Autodesk Fusion 360 part; units mm, degrees
note: some values were not read from the file. Chosen so that the rebuilt part matches the saved one: which bodies a step acts on; which face or edge a step refers to. Set by a fixed rule: which sketch regions a step uses.
(part 3 of 3)
sketch "Sketch1" plane through (0, 0, 0) normal (0, 0, 1) x (1, 0, 0)
  line L0 (-92, 39) -> (92, 39)
  line L1 (92, 39) -> (92, -39)
  line L2 (92, -39) -> (-92, -39)
  line L3 (-92, -39) -> (-92, 39)
  line L4 (-92, 39) -> (92, -39) construction
  line L5 (92, 39) -> (-92, -39) construction
  dimension "d1" = 184
  dimension "d2" = 78
  constraint horizontal L0
  constraint perpendicular L0 L1
  constraint parallel L0 L2
  constraint parallel L1 L3
  constraint coincident L4 origin
  constraint coincident L5 origin
  measures "d1" distance of L1.end L2.end
  measures "d2" distance of L0.end L1.end
extrude "Extrude1" add sketch "Sketch1" along normal blind 6
sketch "Sketch2" plane through (0, 0, 6) normal (0, 0, 1) x (-1, 0, 0)
  line L0 (92, 39) -> (-92, 39)
  line L1 (-92, 39) -> (-92, -39)
  line L2 (-92, -39) -> (92, -39)
  line L3 (92, -39) -> (92, 39)
  line L4 (87, -34) -> (81, -34)
  line L5 (81, -34) -> (81, -29)
  line L6 (81, -29) -> (87, -29)
  line L7 (87, -29) -> (87, -34)
  dimension "d5" = 6
  dimension "d6" = 5
  constraint horizontal L4
  constraint vertical L5
  constraint horizontal L6
  constraint vertical L7
  measures "d5" distance of L4.start L4.end
  measures "d6" distance of L4.start L6.end
extrude "Extrude2" cut sketch "Sketch2" against normal blind 6 contours L4 L5 L6 L7
pattern_linear "R-Pattern1" count 6 spacing 12.6 along (0, -1, 0) count 6 spacing 33.4 along (1, 0, 0) of "Extrude2"
sketch "Sketch3" plane through (0, 0, 6) normal (0, 0, 1) x (-1, 0, 0)
  line L0 (-86, 29) -> (-86, 34)
  line L1 (-86, 34) -> (-80, 34)
  line L2 (-80, 34) -> (-80, 29)
  line L3 (-80, 29) -> (-86, 29)
  line L4 (-86, 16.4) -> (-86, 21.4)
  line L5 (-86, 21.4) -> (-80, 21.4)
  line L6 (-80, 21.4) -> (-80, 16.4)
  line L7 (-80, 16.4) -> (-86, 16.4)
  line L8 (-86, 3.8) -> (-86, 8.8)
  line L9 (-86, 8.8) -> (-80, 8.8)
  line L10 (-80, 8.8) -> (-80, 3.8)
  line L11 (-80, 3.8) -> (-86, 3.8)
  line L12 (-86, -8.8) -> (-86, -3.8)
  line L13 (-86, -3.8) -> (-80, -3.8)
  line L14 (-80, -3.8) -> (-80, -8.8)
  line L15 (-80, -8.8) -> (-86, -8.8)
  line L16 (-86, -21.4) -> (-86, -16.4)
  line L17 (-86, -16.4) -> (-80, -16.4)
  line L18 (-80, -16.4) -> (-80, -21.4)
  line L19 (-80, -21.4) -> (-86, -21.4)
  line L20 (-86, -34) -> (-86, -29)
  line L21 (-86, -29) -> (-80, -29)
  line L22 (-80, -29) -> (-80, -34)
  line L23 (-80, -34) -> (-86, -34)
  line L24 (-52.6, 29) -> (-52.6, 34)
  line L25 (-52.6, 34) -> (-46.6, 34)
  line L26 (-46.6, 34) -> (-46.6, 29)
  line L27 (-46.6, 29) -> (-52.6, 29)
  line L28 (-52.6, 16.4) -> (-52.6, 21.4)
  line L29 (-52.6, 21.4) -> (-46.6, 21.4)
  line L30 (-46.6, 21.4) -> (-46.6, 16.4)
  line L31 (-46.6, 16.4) -> (-52.6, 16.4)
  line L32 (-52.6, 3.8) -> (-52.6, 8.8)
  line L33 (-52.6, 8.8) -> (-46.6, 8.8)
  line L34 (-46.6, 8.8) -> (-46.6, 3.8)
  line L35 (-46.6, 3.8) -> (-52.6, 3.8)
  line L36 (-52.6, -8.8) -> (-52.6, -3.8)
  line L37 (-52.6, -3.8) -> (-46.6, -3.8)
  line L38 (-46.6, -3.8) -> (-46.6, -8.8)
  line L39 (-46.6, -8.8) -> (-52.6, -8.8)
  line L40 (-52.6, -21.4) -> (-52.6, -16.4)
  line L41 (-52.6, -16.4) -> (-46.6, -16.4)
  line L42 (-46.6, -16.4) -> (-46.6, -21.4)
  line L43 (-46.6, -21.4) -> (-52.6, -21.4)
  line L44 (-52.6, -34) -> (-52.6, -29)
  line L45 (-52.6, -29) -> (-46.6, -29)
  line L46 (-46.6, -29) -> (-46.6, -34)
  line L47 (-46.6, -34) -> (-52.6, -34)
  line L48 (-19.2, 29) -> (-19.2, 34)
  line L49 (-19.2, 34) -> (-13.2, 34)
  line L50 (-13.2, 34) -> (-13.2, 29)
  line L51 (-13.2, 29) -> (-19.2, 29)
  line L52 (-19.2, 16.4) -> (-19.2, 21.4)
  line L53 (-19.2, 21.4) -> (-13.2, 21.4)
  line L54 (-13.2, 21.4) -> (-13.2, 16.4)
  line L55 (-13.2, 16.4) -> (-19.2, 16.4)
  line L56 (-19.2, 3.8) -> (-19.2, 8.8)
  line L57 (-19.2, 8.8) -> (-13.2, 8.8)
  line L58 (-13.2, 8.8) -> (-13.2, 3.8)
  line L59 (-13.2, 3.8) -> (-19.2, 3.8)
  line L60 (-19.2, -8.8) -> (-19.2, -3.8)
  line L61 (-19.2, -3.8) -> (-13.2, -3.8)
  line L62 (-13.2, -3.8) -> (-13.2, -8.8)
  line L63 (-13.2, -8.8) -> (-19.2, -8.8)
  line L64 (-19.2, -21.4) -> (-19.2, -16.4)
  line L65 (-19.2, -16.4) -> (-13.2, -16.4)
  line L66 (-13.2, -16.4) -> (-13.2, -21.4)
  line L67 (-13.2, -21.4) -> (-19.2, -21.4)
  line L68 (-19.2, -34) -> (-19.2, -29)
  line L69 (-19.2, -29) -> (-13.2, -29)
  line L70 (-13.2, -29) -> (-13.2, -34)
  line L71 (-13.2, -34) -> (-19.2, -34)
  line L72 (14.2, 29) -> (14.2, 34)
  line L73 (14.2, 34) -> (20.2, 34)
  line L74 (20.2, 34) -> (20.2, 29)
  line L75 (20.2, 29) -> (14.2, 29)
  line L76 (14.2, 16.4) -> (14.2, 21.4)
  line L77 (14.2, 21.4) -> (20.2, 21.4)
  line L78 (20.2, 21.4) -> (20.2, 16.4)
  line L79 (20.2, 16.4) -> (14.2, 16.4)
  line L80 (14.2, 3.8) -> (14.2, 8.8)
  line L81 (14.2, 8.8) -> (20.2, 8.8)
  line L82 (20.2, 8.8) -> (20.2, 3.8)
  line L83 (20.2, 3.8) -> (14.2, 3.8)
  line L84 (14.2, -8.8) -> (14.2, -3.8)
  line L85 (14.2, -3.8) -> (20.2, -3.8)
  line L86 (20.2, -3.8) -> (20.2, -8.8)
  line L87 (20.2, -8.8) -> (14.2, -8.8)
  line L88 (14.2, -21.4) -> (14.2, -16.4)
  line L89 (14.2, -16.4) -> (20.2, -16.4)
  line L90 (20.2, -16.4) -> (20.2, -21.4)
  line L91 (20.2, -21.4) -> (14.2, -21.4)
  line L92 (14.2, -34) -> (14.2, -29)
  line L93 (14.2, -29) -> (20.2, -29)
  line L94 (20.2, -29) -> (20.2, -34)
  line L95 (20.2, -34) -> (14.2, -34)
  line L96 (47.6, 29) -> (47.6, 34)
  line L97 (47.6, 34) -> (53.6, 34)
  line L98 (53.6, 34) -> (53.6, 29)
  line L99 (53.6, 29) -> (47.6, 29)
  line L100 (47.6, 16.4) -> (47.6, 21.4)
  line L101 (47.6, 21.4) -> (53.6, 21.4)
  line L102 (53.6, 21.4) -> (53.6, 16.4)
  line L103 (53.6, 16.4) -> (47.6, 16.4)
  line L104 (47.6, 3.8) -> (47.6, 8.8)
  line L105 (47.6, 8.8) -> (53.6, 8.8)
  line L106 (53.6, 8.8) -> (53.6, 3.8)
  line L107 (53.6, 3.8) -> (47.6, 3.8)
  line L108 (47.6, -8.8) -> (47.6, -3.8)
  line L109 (47.6, -3.8) -> (53.6, -3.8)
  line L110 (53.6, -3.8) -> (53.6, -8.8)
  line L111 (53.6, -8.8) -> (47.6, -8.8)
  line L112 (47.6, -21.4) -> (47.6, -16.4)
  line L113 (47.6, -16.4) -> (53.6, -16.4)
  line L114 (53.6, -16.4) -> (53.6, -21.4)
  line L115 (53.6, -21.4) -> (47.6, -21.4)
  line L116 (47.6, -34) -> (47.6, -29)
  line L117 (47.6, -29) -> (53.6, -29)
  line L118 (53.6, -29) -> (53.6, -34)
  line L119 (53.6, -34) -> (47.6, -34)
  line L120 (81, 29) -> (81, 34)
  line L121 (81, 34) -> (87, 34)
  line L122 (87, 34) -> (87, 29)
  line L123 (87, 29) -> (81, 29)
  line L124 (81, 16.4) -> (81, 21.4)
  line L125 (81, 21.4) -> (87, 21.4)
  line L126 (87, 21.4) -> (87, 16.4)
  line L127 (87, 16.4) -> (81, 16.4)
  line L128 (81, 3.8) -> (81, 8.8)
  line L129 (81, 8.8) -> (87, 8.8)
  line L130 (87, 8.8) -> (87, 3.8)
  line L131 (87, 3.8) -> (81, 3.8)
  line L132 (81, -8.8) -> (81, -3.8)
  line L133 (81, -3.8) -> (87, -3.8)
  line L134 (87, -3.8) -> (87, -8.8)
  line L135 (87, -8.8) -> (81, -8.8)
  line L136 (81, -21.4) -> (81, -16.4)
  line L137 (81, -16.4) -> (87, -16.4)
  line L138 (87, -16.4) -> (87, -21.4)
  line L139 (87, -21.4) -> (81, -21.4)
  line L140 (81, -34) -> (81, -29)
  line L141 (81, -29) -> (87, -29)
  line L142 (87, -29) -> (87, -34)
  line L143 (87, -34) -> (81, -34)
  line L144 (92, 39) -> (-92, 39)
  line L145 (-92, 39) -> (-92, -39)
  line L146 (-92, -39) -> (92, -39)
  line L147 (92, -39) -> (92, 39)
  line L148 (53.6, -34) -> (81, -34) construction
  line L149 (67.3, -34) -> (67.3, 39) construction
  line L150 (70, -34) -> (65, -34)
  line L151 (65, -34) -> (65, -28)
  line L152 (65, -28) -> (70, -28)
  line L153 (70, -28) -> (70, -34)
  dimension "d13" = 6
  dimension "d14" = 5
  constraint coincident L118.end L119.start
  constraint coincident L140.start L143.end
  constraint midpoint L148 L149.start
  constraint coincident L144 L149.end
  constraint perpendicular L144 L149
  constraint horizontal L150
  constraint vertical L151
  constraint horizontal L152
  constraint vertical L153
  constraint coincident L148 L150.start
  measures "d13" distance of L150.start L152.end
  measures "d14" distance of L151 L153
extrude "Extrude3" cut sketch "Sketch3" against normal blind 6 contours L150 L151 L152 L153
pattern_linear "R-Pattern2" count 5 spacing 15.5 along (0, -1, 0) count 5 spacing 33.75 along (1, 0, 0) of "Extrude3"
fillet "Fillet1" radius 3 1 edges at (-92, -39, 3)
fillet "Fillet1" radius 3 3 edges at (-92, 39, 3) (92, 39, 3) (92, -39, 3)
sketch "Sketch4" plane through (0, 0, 6) normal (0, 0, 1) x (-1, 0, 0)
  line L0 (-70, 28) -> (-70, 34)
  line L1 (-70, 34) -> (-65, 34)
  line L2 (-65, 34) -> (-65, 28)
  line L3 (-65, 28) -> (-70, 28)
  line L4 (-70, 12.5) -> (-70, 18.5)
  line L5 (-70, 18.5) -> (-65, 18.5)
  line L6 (-65, 18.5) -> (-65, 12.5)
  line L7 (-65, 12.5) -> (-70, 12.5)
  line L8 (-70, -3) -> (-70, 3)
  line L9 (-70, 3) -> (-65, 3)
  line L10 (-65, 3) -> (-65, -3)
  line L11 (-65, -3) -> (-70, -3)
  line L12 (-70, -18.5) -> (-70, -12.5)
  line L13 (-70, -12.5) -> (-65, -12.5)
  line L14 (-65, -12.5) -> (-65, -18.5)
  line L15 (-65, -18.5) -> (-70, -18.5)
  line L16 (-70, -34) -> (-70, -28)
  line L17 (-70, -28) -> (-65, -28)
  line L18 (-65, -28) -> (-65, -34)
  line L19 (-65, -34) -> (-70, -34)
  line L20 (-36.25, 28) -> (-36.25, 34)
  line L21 (-36.25, 34) -> (-31.25, 34)
  line L22 (-31.25, 34) -> (-31.25, 28)
  line L23 (-31.25, 28) -> (-36.25, 28)
  line L24 (-36.25, 12.5) -> (-36.25, 18.5)
  line L25 (-36.25, 18.5) -> (-31.25, 18.5)
  line L26 (-31.25, 18.5) -> (-31.25, 12.5)
  line L27 (-31.25, 12.5) -> (-36.25, 12.5)
  line L28 (-36.25, -3) -> (-36.25, 3)
  line L29 (-36.25, 3) -> (-31.25, 3)
  line L30 (-31.25, 3) -> (-31.25, -3)
  line L31 (-31.25, -3) -> (-36.25, -3)
  line L32 (-36.25, -18.5) -> (-36.25, -12.5)
  line L33 (-36.25, -12.5) -> (-31.25, -12.5)
  line L34 (-31.25, -12.5) -> (-31.25, -18.5)
  line L35 (-31.25, -18.5) -> (-36.25, -18.5)
  line L36 (-36.25, -34) -> (-36.25, -28)
  line L37 (-36.25, -28) -> (-31.25, -28)
  line L38 (-31.25, -28) -> (-31.25, -34)
  line L39 (-31.25, -34) -> (-36.25, -34)
  line L40 (-2.5, 28) -> (-2.5, 34)
  line L41 (-2.5, 34) -> (2.5, 34)
  line L42 (2.5, 34) -> (2.5, 28)
  line L43 (2.5, 28) -> (-2.5, 28)
  line L44 (-2.5, 12.5) -> (-2.5, 18.5)
  line L45 (-2.5, 18.5) -> (2.5, 18.5)
  line L46 (2.5, 18.5) -> (2.5, 12.5)
  line L47 (2.5, 12.5) -> (-2.5, 12.5)
  line L48 (-2.5, -3) -> (-2.5, 3)
  line L49 (-2.5, 3) -> (2.5, 3)
  line L50 (2.5, 3) -> (2.5, -3)
  line L51 (2.5, -3) -> (-2.5, -3)
  line L52 (-2.5, -18.5) -> (-2.5, -12.5)
  line L53 (-2.5, -12.5) -> (2.5, -12.5)
  line L54 (2.5, -12.5) -> (2.5, -18.5)
  line L55 (2.5, -18.5) -> (-2.5, -18.5)
  line L56 (-2.5, -34) -> (-2.5, -28)
  line L57 (-2.5, -28) -> (2.5, -28)
  line L58 (2.5, -28) -> (2.5, -34)
  line L59 (2.5, -34) -> (-2.5, -34)
  line L60 (31.25, 28) -> (31.25, 34)
  line L61 (31.25, 34) -> (36.25, 34)
  line L62 (36.25, 34) -> (36.25, 28)
  line L63 (36.25, 28) -> (31.25, 28)
  line L64 (31.25, 12.5) -> (31.25, 18.5)
  line L65 (31.25, 18.5) -> (36.25, 18.5)
  line L66 (36.25, 18.5) -> (36.25, 12.5)
  line L67 (36.25, 12.5) -> (31.25, 12.5)
  line L68 (31.25, -3) -> (31.25, 3)
  line L69 (31.25, 3) -> (36.25, 3)
  line L70 (36.25, 3) -> (36.25, -3)
  line L71 (36.25, -3) -> (31.25, -3)
  line L72 (31.25, -18.5) -> (31.25, -12.5)
  line L73 (31.25, -12.5) -> (36.25, -12.5)
  line L74 (36.25, -12.5) -> (36.25, -18.5)
  line L75 (36.25, -18.5) -> (31.25, -18.5)
  line L76 (31.25, -34) -> (31.25, -28)
  line L77 (31.25, -28) -> (36.25, -28)
  line L78 (36.25, -28) -> (36.25, -34)
  line L79 (36.25, -34) -> (31.25, -34)
  line L80 (65, 28) -> (65, 34)
  line L81 (65, 34) -> (70, 34)
  line L82 (70, 34) -> (70, 28)
  line L83 (70, 28) -> (65, 28)
  line L84 (65, 12.5) -> (65, 18.5)
  line L85 (65, 18.5) -> (70, 18.5)
  line L86 (70, 18.5) -> (70, 12.5)
  line L87 (70, 12.5) -> (65, 12.5)
  line L88 (65, -3) -> (65, 3)
  line L89 (65, 3) -> (70, 3)
  line L90 (70, 3) -> (70, -3)
  line L91 (70, -3) -> (65, -3)
  line L92 (65, -18.5) -> (65, -12.5)
  line L93 (65, -12.5) -> (70, -12.5)
  line L94 (70, -12.5) -> (70, -18.5)
  line L95 (70, -18.5) -> (65, -18.5)
  line L96 (65, -34) -> (65, -28)
  line L97 (65, -28) -> (70, -28)
  line L98 (70, -28) -> (70, -34)
  line L99 (70, -34) -> (65, -34)
  line L100 (-86, 29) -> (-86, 34)
  line L101 (-86, 34) -> (-80, 34)
  line L102 (-80, 34) -> (-80, 29)
  line L103 (-80, 29) -> (-86, 29)
  line L104 (-86, 16.4) -> (-86, 21.4)
  line L105 (-86, 21.4) -> (-80, 21.4)
  line L106 (-80, 21.4) -> (-80, 16.4)
  line L107 (-80, 16.4) -> (-86, 16.4)
  line L108 (-86, 3.8) -> (-86, 8.8)
  line L109 (-86, 8.8) -> (-80, 8.8)
  line L110 (-80, 8.8) -> (-80, 3.8)
  line L111 (-80, 3.8) -> (-86, 3.8)
  line L112 (-86, -8.8) -> (-86, -3.8)
  line L113 (-86, -3.8) -> (-80, -3.8)
  line L114 (-80, -3.8) -> (-80, -8.8)
  line L115 (-80, -8.8) -> (-86, -8.8)
  line L116 (-86, -21.4) -> (-86, -16.4)
  line L117 (-86, -16.4) -> (-80, -16.4)
  line L118 (-80, -16.4) -> (-80, -21.4)
  line L119 (-80, -21.4) -> (-86, -21.4)
  line L120 (-86, -34) -> (-86, -29)
  line L121 (-86, -29) -> (-80, -29)
  line L122 (-80, -29) -> (-80, -34)
  line L123 (-80, -34) -> (-86, -34)
  line L124 (-52.6, 29) -> (-52.6, 34)
  line L125 (-52.6, 34) -> (-46.6, 34)
  line L126 (-46.6, 34) -> (-46.6, 29)
  line L127 (-46.6, 29) -> (-52.6, 29)
  line L128 (-52.6, 16.4) -> (-52.6, 21.4)
  line L129 (-52.6, 21.4) -> (-46.6, 21.4)
  line L130 (-46.6, 21.4) -> (-46.6, 16.4)
  line L131 (-46.6, 16.4) -> (-52.6, 16.4)
  line L132 (-52.6, 3.8) -> (-52.6, 8.8)
  line L133 (-52.6, 8.8) -> (-46.6, 8.8)
  line L134 (-46.6, 8.8) -> (-46.6, 3.8)
  line L135 (-46.6, 3.8) -> (-52.6, 3.8)
  line L136 (-52.6, -8.8) -> (-52.6, -3.8)
  line L137 (-52.6, -3.8) -> (-46.6, -3.8)
  line L138 (-46.6, -3.8) -> (-46.6, -8.8)
  line L139 (-46.6, -8.8) -> (-52.6, -8.8)
  line L140 (-52.6, -21.4) -> (-52.6, -16.4)
  line L141 (-52.6, -16.4) -> (-46.6, -16.4)
  line L142 (-46.6, -16.4) -> (-46.6, -21.4)
  line L143 (-46.6, -21.4) -> (-52.6, -21.4)
  line L144 (-52.6, -34) -> (-52.6, -29)
  line L145 (-52.6, -29) -> (-46.6, -29)
  line L146 (-46.6, -29) -> (-46.6, -34)
  line L147 (-46.6, -34) -> (-52.6, -34)
  line L148 (-19.2, 29) -> (-19.2, 34)
  line L149 (-19.2, 34) -> (-13.2, 34)
  line L150 (-13.2, 34) -> (-13.2, 29)
  line L151 (-13.2, 29) -> (-19.2, 29)
  line L152 (-19.2, 16.4) -> (-19.2, 21.4)
  line L153 (-19.2, 21.4) -> (-13.2, 21.4)
  line L154 (-13.2, 21.4) -> (-13.2, 16.4)
  line L155 (-13.2, 16.4) -> (-19.2, 16.4)
  line L156 (-19.2, 3.8) -> (-19.2, 8.8)
  line L157 (-19.2, 8.8) -> (-13.2, 8.8)
  line L158 (-13.2, 8.8) -> (-13.2, 3.8)
  line L159 (-13.2, 3.8) -> (-19.2, 3.8)
  line L160 (-19.2, -8.8) -> (-19.2, -3.8)
  line L161 (-19.2, -3.8) -> (-13.2, -3.8)
  line L162 (-13.2, -3.8) -> (-13.2, -8.8)
  line L163 (-13.2, -8.8) -> (-19.2, -8.8)
  line L164 (-19.2, -21.4) -> (-19.2, -16.4)
  line L165 (-19.2, -16.4) -> (-13.2, -16.4)
  line L166 (-13.2, -16.4) -> (-13.2, -21.4)
  line L167 (-13.2, -21.4) -> (-19.2, -21.4)
  line L168 (-19.2, -34) -> (-19.2, -29)
  line L169 (-19.2, -29) -> (-13.2, -29)
  line L170 (-13.2, -29) -> (-13.2, -34)
  line L171 (-13.2, -34) -> (-19.2, -34)
  line L172 (14.2, 29) -> (14.2, 34)
  line L173 (14.2, 34) -> (20.2, 34)
  line L174 (20.2, 34) -> (20.2, 29)
  line L175 (20.2, 29) -> (14.2, 29)
  line L176 (14.2, 16.4) -> (14.2, 21.4)
  line L177 (14.2, 21.4) -> (20.2, 21.4)
  line L178 (20.2, 21.4) -> (20.2, 16.4)
  line L179 (20.2, 16.4) -> (14.2, 16.4)
  line L180 (14.2, 3.8) -> (14.2, 8.8)
  line L181 (14.2, 8.8) -> (20.2, 8.8)
  line L182 (20.2, 8.8) -> (20.2, 3.8)
  line L183 (20.2, 3.8) -> (14.2, 3.8)
  line L184 (14.2, -8.8) -> (14.2, -3.8)
  line L185 (14.2, -3.8) -> (20.2, -3.8)
  line L186 (20.2, -3.8) -> (20.2, -8.8)
  line L187 (20.2, -8.8) -> (14.2, -8.8)
  line L188 (14.2, -21.4) -> (14.2, -16.4)
  line L189 (14.2, -16.4) -> (20.2, -16.4)
  line L190 (20.2, -16.4) -> (20.2, -21.4)
  line L191 (20.2, -21.4) -> (14.2, -21.4)
  line L192 (14.2, -34) -> (14.2, -29)
  line L193 (14.2, -29) -> (20.2, -29)
  line L194 (20.2, -29) -> (20.2, -34)
  line L195 (20.2, -34) -> (14.2, -34)
  line L196 (47.6, 29) -> (47.6, 34)
  line L197 (47.6, 34) -> (53.6, 34)
  line L198 (53.6, 34) -> (53.6, 29)
  line L199 (53.6, 29) -> (47.6, 29)
  line L200 (47.6, 16.4) -> (47.6, 21.4)
  line L201 (47.6, 21.4) -> (53.6, 21.4)
  line L202 (53.6, 21.4) -> (53.6, 16.4)
  line L203 (53.6, 16.4) -> (47.6, 16.4)
  line L204 (47.6, 3.8) -> (47.6, 8.8)
  line L205 (47.6, 8.8) -> (53.6, 8.8)
  line L206 (53.6, 8.8) -> (53.6, 3.8)
  line L207 (53.6, 3.8) -> (47.6, 3.8)
  line L208 (47.6, -8.8) -> (47.6, -3.8)
  line L209 (47.6, -3.8) -> (53.6, -3.8)
  line L210 (53.6, -3.8) -> (53.6, -8.8)
  line L211 (53.6, -8.8) -> (47.6, -8.8)
  line L212 (47.6, -21.4) -> (47.6, -16.4)
  line L213 (47.6, -16.4) -> (53.6, -16.4)
  line L214 (53.6, -16.4) -> (53.6, -21.4)
  line L215 (53.6, -21.4) -> (47.6, -21.4)
  line L216 (47.6, -34) -> (47.6, -29)
  line L217 (47.6, -29) -> (53.6, -29)
  line L218 (53.6, -29) -> (53.6, -34)
  line L219 (53.6, -34) -> (47.6, -34)
  line L220 (81, 29) -> (81, 34)
  line L221 (81, 34) -> (87, 34)
  line L222 (87, 34) -> (87, 29)
  line L223 (87, 29) -> (81, 29)
  line L224 (81, 16.4) -> (81, 21.4)
  line L225 (81, 21.4) -> (87, 21.4)
  line L226 (87, 21.4) -> (87, 16.4)
  line L227 (87, 16.4) -> (81, 16.4)
  line L228 (81, 3.8) -> (81, 8.8)
  line L229 (81, 8.8) -> (87, 8.8)
  line L230 (87, 8.8) -> (87, 3.8)
  line L231 (87, 3.8) -> (81, 3.8)
  line L232 (81, -8.8) -> (81, -3.8)
  line L233 (81, -3.8) -> (87, -3.8)
  line L234 (87, -3.8) -> (87, -8.8)
  line L235 (87, -8.8) -> (81, -8.8)
  line L236 (81, -21.4) -> (81, -16.4)
  line L237 (81, -16.4) -> (87, -16.4)
  line L238 (87, -16.4) -> (87, -21.4)
  line L239 (87, -21.4) -> (81, -21.4)
  line L240 (81, -34) -> (81, -29)
  line L241 (81, -29) -> (87, -29)
  line L242 (87, -29) -> (87, -34)
  line L243 (87, -34) -> (81, -34)
  arc A0 (-89, 39) -> (-92, 36) centre (-89, 36) ccw
  line L244 (-92, 36) -> (-92, -36)
  arc A1 (-92, -36) -> (-89, -39) centre (-89, -36) ccw
  line L245 (-89, -39) -> (89, -39)
  arc A2 (89, -39) -> (92, -36) centre (89, -36) ccw
  line L246 (92, -36) -> (92, 36)
  arc A3 (92, 36) -> (89, 39) centre (89, 36) ccw
  line L247 (89, 39) -> (-89, 39)

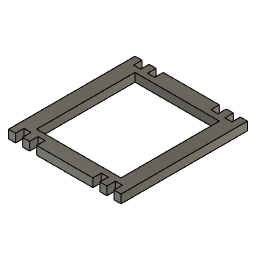
design "Carrier Top Piece"
Autodesk Fusion 360 part; units mm, degrees
sketch "Sketch1" plane through (0, 0, 0) normal (0, 0, 1) x (1, 0, 0)
  line L0 (40, 45) -> (-40, 45)
  line L1 (-40, 45) -> (-40, -45)
  line L2 (-40, -45) -> (40, -45)
  line L3 (40, -45) -> (40, 45)
  line L4 (40, 45) -> (-40, -45) construction
  line L5 (-40, 45) -> (40, -45) construction
  line L6 (30, 35) -> (-30, 35)
  line L7 (-30, 35) -> (-30, -35)
  line L8 (-30, -35) -> (30, -35)
  line L9 (30, -35) -> (30, 35)
  line L10 (30, 35) -> (-30, -35) construction
  line L11 (-30, 35) -> (30, -35) construction
  dimension "d1" = 80
  dimension "d2" = 90
  dimension "d3" = 60
  dimension "d6" = 10
  constraint horizontal L0
  constraint perpendicular L0 L1
  constraint parallel L0 L2
  constraint parallel L1 L3
  constraint coincident L4 origin
  constraint coincident L5 origin
  constraint horizontal L6
  constraint perpendicular L6 L7
  constraint parallel L6 L8
  constraint parallel L7 L9
  constraint coincident L10 origin
  constraint coincident L11 origin
  measures "d1" distance of L1.end L2.end
  measures "d2" distance of L0.end L1.end
  measures "d3" distance of L7.end L8.end
  measures "d6" distance of L0 L6
extrude "Extrude1" add sketch "Sketch1" along normal blind 6
sketch "Sketch2" plane through (0, 0, 6) normal (0, 0, 1) x (-1, 0, 0)
  line L0 (-30, -35) -> (-30, 35)
  line L1 (-30, 35) -> (30, 35)
  line L2 (30, 35) -> (30, -35)
  line L3 (30, -35) -> (-30, -35)
  line L4 (-40, 45) -> (-40, -45)
  line L5 (-40, -45) -> (40, -45)
  line L6 (40, -45) -> (40, 45)
  line L7 (40, 45) -> (-40, 45)
  line L8 (-40, 45) -> (-35, 45) construction
  line L9 (-35, 45) -> (-35, 39) construction
  line L10 (-35, 39) -> (-40, 39) construction
  line L11 (-40, 39) -> (-40, 45) construction
  line L12 (-35, 45) -> (-30, 45) construction
  line L13 (-30, 45) -> (-30, 39) construction
  line L14 (-30, 39) -> (-35, 39) construction
  line L15 (-35, 39) -> (-35, 45) construction
  line L16 (-30, 45) -> (-25, 45) construction
  line L17 (-25, 45) -> (-25, 39) construction
  line L18 (-25, 39) -> (-30, 39) construction
  line L19 (-30, 39) -> (-30, 45) construction
  line L20 (-25, 45) -> (-20, 45) construction
  line L21 (-20, 45) -> (-20, 39) construction
  line L22 (-20, 39) -> (-25, 39) construction
  line L23 (-25, 39) -> (-25, 45) construction
  line L24 (-30, 39) -> (-35, 39)
  line L25 (-35, 39) -> (-35, 45)
  line L26 (-35, 45) -> (-30, 45)
  line L27 (-30, 45) -> (-30, 39)
  line L28 (-20, 39) -> (-25, 39)
  line L29 (-25, 39) -> (-25, 45)
  line L30 (-25, 45) -> (-20, 45)
  line L31 (-20, 45) -> (-20, 39)
  line L32 (40, 45) -> (35, 45) construction
  line L33 (35, 45) -> (35, 39) construction
  line L34 (35, 39) -> (40, 39) construction
  line L35 (40, 39) -> (40, 45) construction
  line L36 (35, 39) -> (30, 39)
  line L37 (30, 39) -> (30, 45)
  line L38 (30, 45) -> (35, 45)
  line L39 (35, 45) -> (35, 39)
  line L40 (30, 39) -> (25, 39) construction
  line L41 (25, 39) -> (25, 45) construction
  line L42 (25, 45) -> (30, 45) construction
  line L43 (30, 45) -> (30, 39) construction
  line L44 (25, 39) -> (20, 39)
  line L45 (20, 39) -> (20, 45)
  line L46 (20, 45) -> (25, 45)
  line L47 (25, 45) -> (25, 39)
  constraint horizontal L8
  constraint vertical L9
  constraint horizontal L10
  constraint vertical L11
  constraint coincident L4.start L7.end
  constraint horizontal L12
  constraint vertical L13
  constraint horizontal L14
  constraint vertical L15
  constraint horizontal L16
  constraint vertical L17
  constraint horizontal L18
  constraint vertical L19
  constraint horizontal L20
  constraint vertical L21
  constraint horizontal L22
  constraint vertical L23
  constraint horizontal L24
  constraint vertical L25
  constraint horizontal L26
  constraint vertical L27
  constraint horizontal L28
  constraint vertical L29
  constraint horizontal L30
  constraint vertical L31
  constraint horizontal L32
  constraint vertical L33
  constraint horizontal L34
  constraint vertical L35
  constraint coincident L6.end L7.start
  constraint horizontal L36
  constraint vertical L37
  constraint horizontal L38
  constraint vertical L39
  constraint coincident L7 L37.end
  constraint horizontal L40
  constraint vertical L41
  constraint horizontal L42
  constraint vertical L43
  constraint coincident L7 L41.end
  constraint horizontal L44
  constraint vertical L45
  constraint horizontal L46
  constraint vertical L47
  constraint coincident L7 L45.end
extrude "Extrude2" cut sketch "Sketch2" against normal blind 6 contours L7 L24 L25 L26 L27 | L7 L28 L29 L30 L31
ref_plane "WorkPlane1" through (0, 0, 0) normal (0, 1, 0) x (0, 0, 1)
ref_plane "WorkPlane2" through (0, 0, 0) normal (1, 0, 0) x (0, 1, 0)
extrude "Extrude3" cut sketch "Sketch2" against normal blind 6 contours L7 L24 L25 L26 L27 | L7 L28 L29 L30 L31 | L7 L36 L37 L38 L39 | L7 L44 L45 L46 L47
mirror "Mirror3" about plane through (0, 0, 0) normal (0, 1, 0) of "Extrude3"
